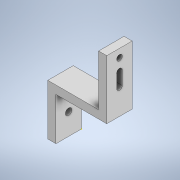
# Autodesk Inventor part: CoilBracketMount
Saved by Autodesk Inventor 2021 (Build 250183000, 183)
## iProperties
Created: 2023-02-03
Part Number: CoilBracketMount
Material: Generic
Document SubType Name: Modeling
Designer: egbrown42
Density: 1 g/cm^3
Appearance: Default
Author: egbrown42
Autodesk Inventor part; units mm, degrees
ref_plane "YZ Plane" through (0, 0, 0) normal (1, 0, 0) x (0, 1, 0)
ref_plane "XZ Plane" through (0, 0, 0) normal (0, 1, 0) x (-1, 0, 0)
ref_plane "XY Plane" through (0, 0, 0) normal (0, 0, 1) x (1, 0, 0)
sketch "Sketch1" plane through (0, 0, 0) normal (0, 0, 1) x (1, 0, 0)
  line L0 (0, 0) -> (0, 50)
  line L1 (0, 50) -> (50, 50)
  line L2 (50, 50) -> (50, 100)
  line L3 (50, 100) -> (58, 100)
  line L4 (58, 100) -> (58, 42)
  line L5 (58, 42) -> (8, 42)
  line L6 (8, 42) -> (8, 0)
  line L7 (8, 0) -> (0, 0)
  dimension "d0" = 50
  dimension "d1" = 50
  dimension "d2" = 50
  dimension "d3" = 8
  dimension "d4" = 58
  dimension "d6" = 50
  constraints: 16 end point, 6 perpendicular, 1 horizontal, 1 vertical
  measures "d0" distance of L0.start L0.end
  measures "d1" distance of L0.end L1.end
  measures "d2" distance of L1.end L2.end
  measures "d3" distance of L2.end L3.end
  measures "d4" distance of L3.end L4.end
  measures "d6" distance of L4.end L5.end
extrude "Extrusion1" add sketch "Sketch1" along normal blind 25
sketch "Sketch2" plane through (58, 42, 0) normal (1, 0, 0) x (0, 0, -1)
  circle A0 centre (-12.5, 50) radius 2.75
  line L0 (0, 58) -> (-25, 58) projected
  line L1 (-25, 0) -> (-25, 58) projected
  point P0 (0, -42)
  dimension "d9" = 5.5
  dimension "d10" = 8
  dimension "d11" = 12.5
  constraints: 1 centre point
  measures "d9" diameter of A0
  measures "d10" distance from line of L0 A0.centre
  measures "d11" distance from line of L1 A0.centre
extrude "Extrusion2" cut sketch "Sketch2" against normal blind 25
sketch "Sketch3" plane through (8, 0, 0) normal (1, 0, 0) x (0, 0, -1)
  point P0 (0, 0)
sketch "Sketch4" plane through (8, 0, 0) normal (1, 0, 0) x (0, 0, -1)
  circle A0 centre (-12.5, 21) radius 3.25
  line L0 (0, 42) -> (-25, 42) projected
  line L1 (0, 0) -> (0, 42) projected
  dimension "d26" = 21
  dimension "d27" = 6.5
  dimension "d28" = 12.5
  constraints: 1 centre point
  measures "d26" distance from line of A0.centre L0
  measures "d27" diameter of A0
  measures "d28" distance from line of A0.centre L1
extrude "Extrusion3" cut sketch "Sketch4" against normal blind 25
sketch "Sketch5" plane through (58, 42, 0) normal (1, 0, 0) x (0, 0, -1)
  circle A0 centre (-12.5, 38.2531) radius 2.75
  line L0 (0, 0) -> (0, 58) projected
  circle A1 centre (-12.5, 24.9243) radius 2.75
  line L1 (-15.25, 38.2531) -> (-15.25, 24.9243)
  line L2 (-9.75, 38.2531) -> (-9.75, 24.9243)
  point P0 (0, -42)
  dimension "d31" = 5.5
  dimension "d32" = 9.75
  dimension "d33" = 5.5
  constraints: 4 end point, 4 point on circle, 2 centre point, 2 tangent
  measures "d31" diameter of A0
  measures "d32" distance edge to line of A0 L0
  measures "d33" diameter of A1
extrude "Extrusion4" cut sketch "Sketch5" against normal blind 58
equation "\"d34\" = d4"
body "Solid1"
